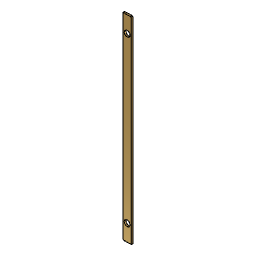
Mount Strip Right (Autodesk Fusion 360 design; units mm, degrees)
Autodesk Fusion 360 part; units mm, degrees
sketch "Sketch1" plane through (0, 0, 0) normal (0, 1, 0) x (1, 0, 0)
  line L0 (5, -120) -> (-5, -120)
  line L1 (-5, -120) -> (-5, 120)
  line L2 (-5, 120) -> (5, 120)
  line L3 (5, 120) -> (5, -120)
  line L4 (5, -120) -> (-5, 120) construction
  line L5 (-5, -120) -> (5, 120) construction
  line L6 (0, -120) -> (0, 120) construction
  circle A0 centre (0, 100) radius 3.5
  circle A1 centre (0, -100) radius 3.5
  dimension "d1" = 240
  dimension "d2" = 10
  dimension "d3" = 7
  dimension "d4" = 7
  dimension "d5" = 200
  dimension "d6" = 20
  constraint perpendicular L0 L1
  constraint parallel L0 L2
  constraint parallel L1 L3
  constraint horizontal L0
  constraint coincident L4 origin
  constraint coincident L5 origin
  constraint midpoint L0 L6.start
  constraint midpoint L2 L6.end
  constraint coincident L6 A0.centre
  constraint coincident L6 A1.centre
  measures "d1" distance of L0.end L1.end
  measures "d2" distance of L1.end L2.end
  measures "d3" diameter of A0
  measures "d4" diameter of A1
  measures "d5" distance of A0.centre A1.centre
  measures "d6" distance of L6.end A0.centre
extrude "Extrude1" add sketch "Sketch1" along normal blind 2
named bodies: "Strip Right"
